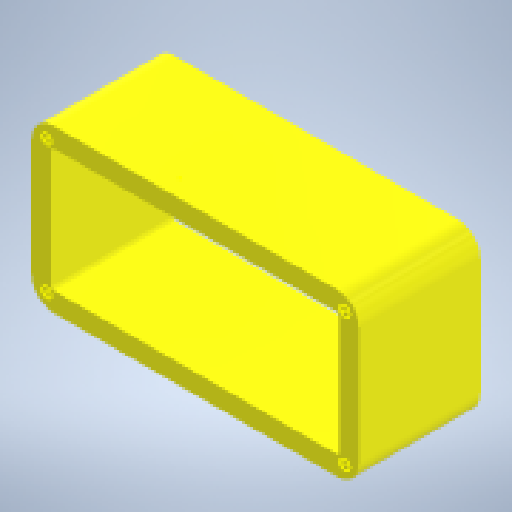
# Autodesk Inventor part: battery hold
Saved by Autodesk Inventor 2024 (Build 280153000, 153)
## iProperties
Created: 2024-01-06
Part Number: battery hold
Material: Generic
Document SubType Name: Modeling
Designer: student
Density: 1 g/cm^3
Appearance: Yellow
Author: student
Autodesk Inventor part; units mm, degrees
ref_plane "YZ Plane" through (0, 0, 0) normal (1, 0, 0) x (0, 1, 0)
ref_plane "XZ Plane" through (0, 0, 0) normal (0, 1, 0) x (-1, 0, 0)
ref_plane "XY Plane" through (0, 0, 0) normal (0, 0, 1) x (1, 0, 0)
sketch "Sketch1" plane through (0, 0, 0) normal (0, 0, 1) x (1, 0, 0)
  line L0 (63.4168, -84.0015) -> (-66.0832, -83.9994) projected
  line L1 (63.4168, -84.0015) -> (81.9168, -84.0018) projected
  line L2 (-67.5831, -82.4994) -> (-67.5821, -20.9994) projected
  arc A0 (-67.5831, -82.4994) -> (-66.0832, -83.9994) centre (-66.0831, -82.4994) ccw projected
  arc A1 (-66.0821, -19.4994) -> (-67.5821, -20.9994) centre (-66.0821, -20.9994) ccw projected
  line L3 (-66.0821, -19.4994) -> (63.4179, -19.5015) projected
  line L4 (64.1679, -20.2516) -> (81.9179, -20.2518) projected
  line L5 (81.9179, -19.5018) -> (63.4179, -19.5015) projected
  arc A2 (83.4179, -21.0019) -> (81.9179, -19.5018) centre (81.9179, -21.0018) ccw projected
  line L6 (83.4176, -39.5019) -> (83.4179, -21.0019) projected
  line L7 (83.4176, -39.5019) -> (83.4172, -64.0019) projected
  line L8 (83.4169, -82.5019) -> (83.4172, -64.0019) projected
  arc A3 (81.9168, -84.0018) -> (83.4169, -82.5019) centre (81.9169, -82.5018) ccw projected
  line L9 (-77.7421, -20.9992) -> (-77.7431, -82.4992)
  arc A4 (-77.7431, -82.4992) -> (-66.0833, -94.1594) centre (-66.0831, -82.4994) ccw
  line L10 (-66.0833, -94.1594) -> (63.4167, -94.1615)
  line L11 (63.4167, -94.1615) -> (81.9167, -94.1618)
  arc A5 (81.9167, -94.1618) -> (93.5769, -82.502) centre (81.9169, -82.5018) ccw
  line L12 (93.5769, -82.502) -> (93.5772, -64.002)
  line L13 (93.5772, -64.002) -> (93.5776, -39.502)
  line L14 (93.5776, -39.502) -> (93.5779, -21.002)
  arc A6 (93.5779, -21.002) -> (81.9181, -9.3418) centre (81.9179, -21.0018) ccw
  line L15 (81.9181, -9.3418) -> (63.4181, -9.3415)
  line L16 (63.4181, -9.3415) -> (-66.0819, -9.3394)
  arc A7 (-66.0819, -9.3394) -> (-77.7421, -20.9992) centre (-66.0821, -20.9994) ccw
  point P0 (0, 0)
  dimension "d0" = 10.16
  constraints: 16 end point, 8 point on circle, 4 centre point, 11 other
  measures "d0" distance between parallel lines of L2 L9
extrude "Extrusion1" add sketch "Sketch1" along normal blind 63.5
sketch "Sketch2" plane through (0, 0, 63.5) normal (0, 0, 1) x (1, 0, 0)
  circle A0 centre (-70.1221, -16.9594) radius 2.54 projected
  circle A1 centre (85.9579, -16.9619) radius 2.54 projected
  circle A2 centre (85.9568, -86.5419) radius 2.54 projected
  circle A3 centre (-70.1232, -86.5394) radius 2.54 projected
  point P0 (0, 0)
hole "Hole1" at (-70.1221, -16.9594, 63.5) at (-70.1232, -86.5394, 63.5) at (85.9579, -16.9619, 63.5) at (85.9568, -86.5419, 63.5) direction (0, 0, -1) diameter 5.08 depth 19.05
body "Solid1"
